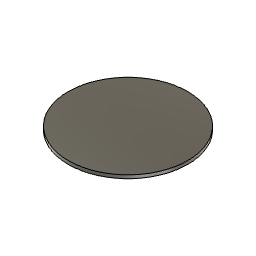
wheel_attachment (Autodesk Fusion 360 design; units mm, degrees)
Autodesk Fusion 360 part; units mm, degrees
cylinder "CylinderPrimitive1" add diameter 72 height 2 placed x (1, 0, 0) y (0, 1, 0) z (0, 0, 1) at (-100, 75, 0)
